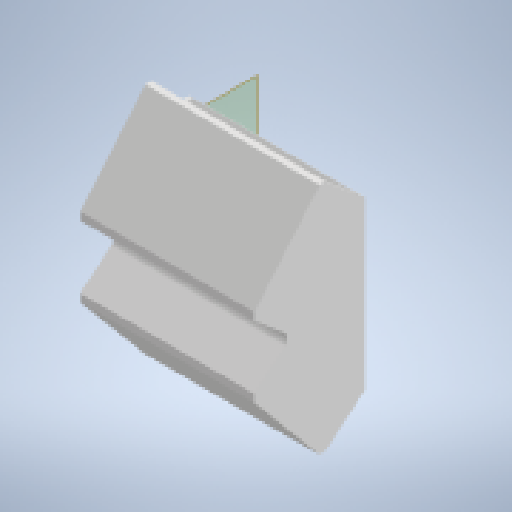
# Autodesk Inventor part: BatterMountv1
Saved by Autodesk Inventor 2023 (Build 270158030, 158C)
## iProperties
Created: 2024-03-25
Part Number: BatterMountv1
Material: Generic
Document SubType Name: Modeling
Designer: lvrectanus0
Density: 1 g/cm^3
Appearance: Default
Author: lvrectanus0
Autodesk Inventor part; units mm, degrees
ref_plane "YZ Plane" through (0, 0, 0) normal (1, 0, 0) x (0, 1, 0)
ref_plane "XZ Plane" through (0, 0, 0) normal (0, 1, 0) x (-1, 0, 0)
ref_plane "XY Plane" through (0, 0, 0) normal (0, 0, 1) x (1, 0, 0)
ref_plane "Work Plane1" through (-37.1475, -26.67, 0) normal (-1, 0, 0) x (0, 0, 1)
sketch "Sketch1" plane through (-37.1475, -26.67, 0) normal (-1, 0, 0) x (0, 0, 1)
  line L0 (-8, 23.8125) -> (-8, 9.525) projected
  line L1 (-8, 9.525) -> (-20.7, 9.525) projected
  ellipse E0 centre (-20.7, 16.6688) end of major axis (-20.7, 23.8125) minor radius 2.54 (-20.7, 23.8125) -> (-20.7, 9.525) ccw projected
  line L2 (-20.7, 23.8125) -> (-8, 23.8125) projected
  ellipse E1 centre (-20.7, 45.2438) end of major axis (-20.7, 50.8) minor radius 2.54 (-20.7, 50.8) -> (-20.7, 39.6875) ccw projected
  line L3 (-20.7, 50.8) -> (-8, 50.8) projected
  line L4 (-8, 50.8) -> (-8, 39.6875) projected
  line L5 (-8, 39.6875) -> (-20.7, 39.6875) projected
  line L6 (0, 53.34) -> (0, 0) projected
  line L7 (0, 53.34) -> (-27.05, 53.34) projected
  line L8 (-27.05, 0) -> (-27.05, 53.34) projected
  line L9 (0, 0) -> (-27.05, 0) projected
  line L10 (0, 0) -> (0, -8.89)
  line L11 (0, -8.89) -> (17.0253, -23.176)
  line L12 (17.0253, -23.176) -> (19.5653, -23.176)
  line L13 (19.5653, -23.176) -> (47.3209, 9.9018)
  line L14 (19.5653, -23.176) -> (62.7453, -23.176) construction
  line L15 (47.3209, 9.9018) -> (47.3209, 12.4418)
  line L16 (47.3209, 12.4418) -> (30.2956, 26.7278) construction
  line L17 (0, -8.89) -> (29.8869, 26.7278) construction
  line L18 (0, -8.89) -> (46.4957, -8.89) construction
  line L19 (30.2956, 26.7278) -> (29.8869, 26.7278) construction
  line L20 (0, 26.67) -> (56.4036, 26.67) construction
  line L21 (47.3209, 12.4418) -> (47.3209, 26.67)
  line L22 (0, 0) -> (0, 26.67)
  line L23 (0, 53.34) -> (0, 62.23)
  line L24 (0, 62.23) -> (17.0253, 76.516)
  line L25 (17.0253, 76.516) -> (19.5653, 76.516)
  line L26 (19.5653, 76.516) -> (47.3209, 43.4382)
  line L27 (19.5653, 76.516) -> (62.7453, 76.516) construction
  line L28 (47.3209, 43.4382) -> (47.3209, 40.8982)
  line L29 (47.3209, 40.8982) -> (30.2956, 26.6122) construction
  line L30 (0, 62.23) -> (29.8869, 26.6122) construction
  line L31 (0, 62.23) -> (46.4957, 62.23) construction
  line L32 (30.2956, 26.6122) -> (29.8869, 26.6122) construction
  line L33 (47.3209, 40.8982) -> (47.3209, 26.67)
  line L34 (0, 53.34) -> (0, 26.67)
  dimension "d0" = 8.89
  dimension "d1" = 22.225
  dimension "d2" = 130
  dimension "d3" = 2.54
  dimension "d4" = 43.18
  dimension "d5" = 50
  dimension "d6" = 2.54
  dimension "d7" = 140
  dimension "d9" = 130
  dimension "d10" = 50
  constraints: 50 end point, 9 symmetric about line, 5 horizontal, 3 equal length, 3 vertical, 2 perpendicular, 1 horizontal alignment, 1 point on line, 2 other
  measures "d0" distance of L6.end L10.end
  measures "d1" distance of L10.end L11.end
  measures "d2" angle of L11 L10
  measures "d3" distance of L11.end L12.end
  measures "d4" distance of L12.end L13.end
  measures "d5" angle of L14 L13
  measures "d6" distance of L13.end L15.end
  measures "d7" angle of L15 L13
  measures "d9" angle of L16 L15
  measures "d10" angle of L18 L17
ref_plane "Work Plane2" through (37.1475, -26.67, -27.05) normal (1, 0, 0) x (0, 1, 0)
extrude "Extrusion1" add sketch "Sketch1" against normal up to surface (74.295 mm away) contours L23 L24 L25 L26 L28 L33 L21 L15 L13 L12 L11 L10 L6
sketch "Sketch2" plane through (-37.1475, -49.846, 17.0253) normal (0, -0.7660444, -0.6427876) x (1, 0, 0)
  line L0 (74.295, -22.225) -> (74.295, 0) projected
  line L1 (0, 0) -> (74.295, 0) projected
  line L2 (0, -22.225) -> (0, 0) projected
  line L3 (0, -22.225) -> (74.295, -22.225) projected
  line L4 (72.7075, -20.6375) -> (72.7075, -1.5875)
  line L5 (72.7075, -1.5875) -> (1.5875, -1.5875)
  line L6 (1.5875, -1.5875) -> (1.5875, -20.6375)
  line L7 (1.5875, -20.6375) -> (72.7075, -20.6375)
  point P0 (37.1475, -45.0825)
  dimension "d13" = 19.05
  constraints: 8 end point, 3 other
  measures "d13" distance between parallel lines of L5 L7
sketch "Sketch3" plane through (-37.1475, 35.56, 0) normal (0, 0.7660444, -0.6427876) x (1, 0, 0)
  line L0 (74.295, -22.225) -> (74.295, 0) projected
  line L1 (0, 0) -> (74.295, 0) projected
  line L2 (0, -22.225) -> (0, 0) projected
  line L3 (0, -22.225) -> (74.295, -22.225) projected
  line L4 (72.7075, -1.5875) -> (72.7075, -20.6375)
  line L5 (72.7075, -20.6375) -> (1.5875, -20.6375)
  line L6 (1.5875, -20.6375) -> (1.5875, -1.5875)
  line L7 (1.5875, -1.5875) -> (72.7075, -1.5875)
  point P0 (37.1475, 22.8575)
  dimension "d14" = 19.05
  constraints: 8 end point, 3 other
  measures "d14" distance between parallel lines of L5 L7
extrude "Extrusion2" cut sketch "Sketch2" against normal blind 44.45 contours L7 L6 L5 L4
extrude "Extrusion3" cut sketch "Sketch3" against normal blind 44.45 contours L4 L5 L6 L7
sketch "Sketch4" plane through (-37.1475, -26.67, 0) normal (-1, 0, 0) x (0, 0, 1)
  line L0 (19.5653, -23.176) -> (47.3209, 9.9018) projected
  line L1 (47.3209, 43.4382) -> (19.5653, 76.516) projected
  line L2 (19.5653, -23.176) -> (47.3209, 9.9018) projected
  line L3 (47.3209, 43.4382) -> (19.5653, 76.516) projected
  line L4 (0, -8.89) -> (17.0253, -23.176) projected
  line L5 (17.0253, -23.176) -> (19.5653, -23.176) projected
  line L6 (19.5653, -23.176) -> (47.3209, 9.9018) projected
  line L7 (47.3209, 9.9018) -> (47.3209, 43.4382) projected
  line L8 (47.3209, 43.4382) -> (19.5653, 76.516) projected
  line L9 (19.5653, 76.516) -> (17.0253, 76.516) projected
  line L10 (17.0253, 76.516) -> (0, 62.23) projected
  line L11 (0, 62.23) -> (0, -8.89) projected
  line L12 (1.2161, -9.9104) -> (15.8092, -22.1555) projected
  line L13 (1.2161, -9.9104) -> (29.788, 24.1403) projected
  line L14 (29.788, 24.1403) -> (44.3812, 11.8951) projected
  line L15 (15.8092, -22.1555) -> (44.3812, 11.8951) projected
  line L16 (15.8092, 75.4955) -> (1.2161, 63.2504) projected
  line L17 (15.8092, 75.4955) -> (44.3812, 41.4449) projected
  line L18 (44.3812, 41.4449) -> (29.788, 29.1997) projected
  line L19 (1.2161, 63.2504) -> (29.788, 29.1997) projected
  line L20 (47.3209, 9.9018) -> (27.3374, 26.67)
  line L21 (27.3374, 26.67) -> (47.3209, 43.4382)
  line L22 (47.3209, 13.2176) -> (31.2889, 26.67)
  line L23 (31.2889, 26.67) -> (47.3209, 40.1224)
  line L24 (47.3209, 9.9018) -> (47.3209, 43.4382) projected
  line L25 (47.3209, 9.9018) -> (47.3209, 43.4382)
  point P0 (0, 26.67)
  point P1 (47.3209, 26.67)
  point P2 (47.3209, 26.67)
  point P3 (47.3209, 13.2176)
  dimension "d20" = 2.54
  constraints: 10 end point, 2 horizontal alignment, 2 midpoint, 2 point on line, 1 collinear, 1 parallel, 1 other
  measures "d20" distance between parallel lines of L20 L22
extrude "Extrusion4" cut sketch "Sketch4" against normal through all contours L22 L23 L7
fillet "Fillet1" radius 3.175 1 edges at (0, 0, 31.2889)
sketch "Sketch5" plane through (-37.1475, -35.56, 0) normal (0, 0, -1) x (-1, 0, 0)
  line L0 (-68.8975, 30.575) -> (-72.7075, 30.575) projected
  arc A0 (-68.8975, 22.765) -> (-68.8975, 30.575) centre (-68.8975, 26.67) ccw projected
  line L1 (-72.7075, 22.765) -> (-68.8975, 22.765) projected
  line L2 (-72.7075, 22.765) -> (-72.7075, 8.89) projected
  arc A1 (-72.7075, 8.89) -> (-71.4375, 7.62) centre (-71.4375, 8.89) ccw projected
  line L3 (-71.4375, 7.62) -> (-22.0025, 7.62) projected
  line L4 (-22.0025, 11.43) -> (-22.0025, 7.62) projected
  arc A2 (-14.1925, 11.43) -> (-22.0025, 11.43) centre (-18.0975, 11.43) ccw projected
  line L5 (-14.1925, 7.62) -> (-14.1925, 11.43) projected
  line L6 (-14.1925, 7.62) -> (-2.8575, 7.62) projected
  arc A3 (-2.8575, 7.62) -> (-1.5875, 8.89) centre (-2.8575, 8.89) ccw projected
  line L7 (-1.5875, 8.89) -> (-1.5875, 62.23) projected
  arc A4 (-1.5875, 62.23) -> (-2.8575, 63.5) centre (-2.8575, 62.23) ccw projected
  line L8 (-2.8575, 63.5) -> (-12.9225, 63.5) projected
  line L9 (-12.9225, 59.69) -> (-12.9225, 63.5) projected
  arc A5 (-20.7325, 59.69) -> (-12.9225, 59.69) centre (-16.8275, 59.69) ccw projected
  line L10 (-20.7325, 63.5) -> (-20.7325, 59.69) projected
  line L11 (-20.7325, 63.5) -> (-71.4375, 63.5) projected
  arc A6 (-71.4375, 63.5) -> (-72.7075, 62.23) centre (-71.4375, 62.23) ccw projected
  line L12 (-72.7075, 62.23) -> (-72.7075, 58.515) projected
  line L13 (-68.8975, 58.515) -> (-72.7075, 58.515) projected
  arc A7 (-68.8975, 50.705) -> (-68.8975, 58.515) centre (-68.8975, 54.61) ccw projected
  line L14 (-72.7075, 50.705) -> (-68.8975, 50.705) projected
  line L15 (-72.7075, 50.705) -> (-72.7075, 30.575) projected
  circle A8 centre (-18.0975, 11.43) radius 2 projected
  circle A9 centre (-68.8975, 26.67) radius 2 projected
  circle A10 centre (-68.8975, 54.61) radius 2 projected
  circle A11 centre (-16.8275, 59.69) radius 2 projected
  point P0 (-37.1475, 35.56)
extrude "Extrusion5" cut sketch "Sketch5" against normal blind 5.8 contours A8 | A9 | A10 | A11
sketch "Sketch6" plane through (-37.1475, -26.67, 0) normal (-1, 0, 0) x (0, 0, 1)
  line L0 (15.8092, -22.1555) -> (1.2161, -9.9104) projected
  line L1 (1.2161, -9.9104) -> (29.788, 24.1403) projected
  arc A0 (15.8092, -22.1555) -> (1.2161, -9.9104) centre (3.1131, -22.468) ccw
  line L2 (1.2161, 63.2504) -> (29.788, 29.1997) projected
  line L3 (15.8092, 75.4955) -> (44.3812, 41.4449) projected
  arc A1 (1.2161, 63.2504) -> (15.8092, 75.4955) centre (3.1131, 75.808) ccw
  line L4 (15.8092, 75.4955) -> (1.2161, 63.2504) projected
  point P0 (0, 26.67)
  dimension "d26" = 12.7
  dimension "d27" = 12.7
  constraints: 4 point on circle, 2 centre point
  measures "d26" radius of A0
  measures "d27" radius of A1
extrude "Extrusion6" cut sketch "Sketch6" against normal up to surface (1.5875 mm away)
sketch "Sketch7" plane through (-37.1475, -26.67, 0) normal (-1, 0, 0) x (0, 0, 1)
  arc A0 (1.2161, 63.2504) -> (15.8092, 75.4955) centre (3.1131, 75.808) ccw projected
  line L0 (1.2161, 63.2504) -> (0, 62.23) projected
  line L1 (0, 62.23) -> (0, -8.89) projected
  line L2 (0, -8.89) -> (1.2161, -9.9104) projected
  arc A1 (15.8092, -22.1555) -> (1.2161, -9.9104) centre (3.1131, -22.468) ccw projected
  line L3 (15.8092, -22.1555) -> (17.0253, -23.176) projected
  line L4 (17.0253, -23.176) -> (19.5653, -23.176) projected
  line L5 (19.5653, -23.176) -> (47.3209, 9.9018) projected
  line L6 (47.3209, 9.9018) -> (47.3209, 13.2176) projected
  line L7 (47.3209, 13.2176) -> (34.1875, 24.2378) projected
  arc A2 (34.1875, 29.1022) -> (34.1875, 24.2378) centre (36.2284, 26.67) ccw projected
  line L8 (34.1875, 29.1022) -> (47.3209, 40.1224) projected
  line L9 (47.3209, 40.1224) -> (47.3209, 43.4382) projected
  line L10 (47.3209, 43.4382) -> (19.5653, 76.516) projected
  line L11 (19.5653, 76.516) -> (17.0253, 76.516) projected
  line L12 (17.0253, 76.516) -> (15.8092, 75.4955) projected
  line L13 (0.3078, 54.17) -> (0.3078, -0.83) projected
  line L14 (6.35, -0.83) -> (0.3078, -0.83) projected
  line L15 (6.35, 54.17) -> (6.35, -0.83) projected
  line L16 (0.3078, 54.17) -> (6.35, 54.17) projected
  line L17 (17.0253, 76.516) -> (0, 62.23) projected
  line L18 (0, 62.23) -> (6.35, 62.23)
  line L19 (6.35, 62.23) -> (6.35, 55.88)
  line L20 (6.35, 55.88) -> (0, 55.88)
  line L21 (0, 55.88) -> (0, 62.23)
  line L22 (47.3209, 43.4382) -> (19.5653, 76.516) projected
  line L23 (24.4634, 70.6787) -> (19.599, 66.597)
  line L24 (19.599, 66.597) -> (23.6807, 61.7326)
  line L25 (23.6807, 61.7326) -> (28.5451, 65.8143)
  line L26 (24.4634, 70.6787) -> (28.5451, 65.8143)
  line L27 (42.4229, 49.2754) -> (37.5585, 45.1937)
  line L28 (37.5585, 45.1937) -> (33.4768, 50.0581)
  line L29 (33.4768, 50.0581) -> (38.3412, 54.1398)
  line L30 (42.4229, 49.2754) -> (38.3412, 54.1398)
  line L31 (36.2284, 26.67) -> (0, 26.67) construction
  arc A3 (15.8092, -22.1555) -> (1.2161, -9.9104) centre (3.1131, -22.468) ccw
  line L32 (1.2161, -9.9104) -> (0, -8.89)
  line L33 (47.3209, 9.9018) -> (19.5653, -23.176)
  line L34 (19.5653, -23.176) -> (17.0253, -23.176)
  line L35 (17.0253, -23.176) -> (15.8092, -22.1555)
  line L36 (0.3078, -0.83) -> (6.35, -0.83)
  line L37 (17.0253, -23.176) -> (0, -8.89)
  line L38 (0, -8.89) -> (6.35, -8.89)
  line L39 (6.35, -8.89) -> (6.35, -2.54)
  line L40 (6.35, -2.54) -> (0, -2.54)
  line L41 (0, -2.54) -> (0, -8.89)
  line L42 (47.3209, 9.9018) -> (19.5653, -23.176)
  line L43 (24.4634, -17.3387) -> (19.599, -13.257)
  line L44 (19.599, -13.257) -> (23.6807, -8.3926)
  line L45 (23.6807, -8.3926) -> (28.5451, -12.4743)
  line L46 (24.4634, -17.3387) -> (28.5451, -12.4743)
  line L47 (42.4229, 4.0646) -> (37.5585, 8.1463)
  line L48 (37.5585, 8.1463) -> (33.4768, 3.2819)
  line L49 (33.4768, 3.2819) -> (38.3412, -0.7998)
  line L50 (42.4229, 4.0646) -> (38.3412, -0.7998)
  circle A4 centre (3.3289, 13.97) radius 2 projected
  circle A5 centre (3.3289, 39.37) radius 2 projected
  point P0 (0, 55.88)
  point P1 (24.4634, -17.3387)
  point P2 (0, -2.54)
  dimension "d30" = 6.35
  dimension "d31" = 6.35
  dimension "d34" = 6.35
  dimension "d35" = 7.62
  dimension "d36" = 6.35
  dimension "d37" = 6.35
  dimension "d38" = 7.62
  constraints: 64 end point, 12 symmetric about line, 8 point on line, 7 perpendicular, 5 parallel, 2 horizontal, 2 point on circle, 1 centre point, 1 collinear, 1 other
  measures "d30" distance of L19.end L20.end
  measures "d31" distance of L18.end L19.end
  measures "d34" distance of L23.start L23.end
  measures "d35" distance of L10.end L23.start
  measures "d36" distance of L23.end L24.end
  measures "d37" distance of L27.end L28.end
  measures "d38" distance of L27.start L9.end
extrude "Extrusion7" add sketch "Sketch7" along normal blind 6.35 contours L18 L19 L20 L1 | L40 L39 L38 L1 | L10 L25 L24 L23 | L10 L27 L28 L29 | L43 L44 L45 L5 | L49 L48 L47 L5
chamfer "Chamfer1" distance 6.35 angle 45 13 edges at (-37.1475, 20.5646, 39.9907) (-37.1475, 37.1035, 26.1129) (-37.1475, -25.4289, 35.909) (-37.1475, -41.9678, 22.0312) (-37.1475, -37.4948, 21.6398) (-37.1475, -20.9559, 35.5176) (-37.1475, -20.5646, 39.9907) (-37.1475, 20.9559, 35.5176) (-37.1475, 25.4289, 35.909) (-37.1475, 41.9678, 22.0312) (-37.1475, 37.4948, 21.6398) (-37.1475, 32.385, 6.35) (-37.1475, -32.385, 6.35)
sketch "Sketch8" plane through (-43.4975, -26.67, 0) normal (-1, 0, 0) x (0, 0, 1)
  line L0 (6.35, -2.54) -> (0, -2.54) construction
  line L1 (0, -2.54) -> (0, -8.89) construction
  line L2 (0, -8.89) -> (6.35, -8.89) construction
  line L3 (6.35, -8.89) -> (6.35, -2.54) construction
  line L4 (19.599, -13.257) -> (24.4634, -17.3387) construction
  line L5 (24.4634, -17.3387) -> (28.5451, -12.4743) construction
  line L6 (28.5451, -12.4743) -> (23.6807, -8.3926) construction
  line L7 (23.6807, -8.3926) -> (19.599, -13.257) construction
  line L8 (33.4768, 3.2819) -> (38.3412, -0.7998) construction
  line L9 (38.3412, -0.7998) -> (42.4229, 4.0646) construction
  line L10 (42.4229, 4.0646) -> (37.5585, 8.1463) construction
  line L11 (37.5585, 8.1463) -> (33.4768, 3.2819) construction
  line L12 (37.5585, 45.1937) -> (42.4229, 49.2754) construction
  line L13 (42.4229, 49.2754) -> (38.3412, 54.1398) construction
  line L14 (38.3412, 54.1398) -> (33.4768, 50.0581) construction
  line L15 (33.4768, 50.0581) -> (37.5585, 45.1937) construction
  line L16 (23.6807, 61.7326) -> (28.5451, 65.8143) construction
  line L17 (28.5451, 65.8143) -> (24.4634, 70.6787) construction
  line L18 (24.4634, 70.6787) -> (19.599, 66.597) construction
  line L19 (19.599, 66.597) -> (23.6807, 61.7326) construction
  line L20 (6.35, 62.23) -> (0, 62.23) construction
  line L21 (0, 62.23) -> (0, 55.88) construction
  line L22 (0, 55.88) -> (6.35, 55.88) construction
  line L23 (6.35, 55.88) -> (6.35, 62.23) construction
  line L24 (0, -2.54) -> (0, -8.89) construction
  line L25 (6.35, -2.54) -> (0, -2.54) construction
  line L26 (0, -8.89) -> (6.35, -2.54) construction
  line L27 (0, -8.89) -> (6.35, -8.89) construction
  line L28 (6.35, -2.54) -> (6.35, -8.89) construction
  line L29 (6.35, -8.89) -> (0, -2.54) construction
  line L30 (23.6807, -8.3926) -> (19.599, -13.257) construction
  line L31 (28.5451, -12.4743) -> (19.599, -13.257) construction
  line L32 (24.4634, -17.3387) -> (28.5451, -12.4743) construction
  line L33 (19.599, -13.257) -> (24.4634, -17.3387) construction
  line L34 (24.4634, -17.3387) -> (23.6807, -8.3926) construction
  line L35 (33.4768, 3.2819) -> (42.4229, 4.0646) construction
  line L36 (24.5307, 2.4992) -> (33.4768, 3.2819) construction
  line L37 (37.5585, 8.1463) -> (36.7758, 17.0924) construction
  line L38 (37.5585, 8.1463) -> (38.3412, -0.7998) construction
  line L39 (33.4768, 50.0581) -> (37.5585, 45.1937) construction
  line L40 (42.4229, 49.2754) -> (38.3412, 54.1398) construction
  line L41 (37.5585, 45.1937) -> (38.3412, 54.1398) construction
  line L42 (38.3412, 54.1398) -> (42.4229, 49.2754) construction
  line L43 (42.4229, 49.2754) -> (33.4768, 50.0581) construction
  line L44 (23.6807, 61.7326) -> (28.5451, 65.8143) construction
  line L45 (23.6807, 61.7326) -> (24.4634, 70.6787) construction
  line L46 (19.599, 66.597) -> (12.4699, 67.2207) construction
  line L47 (19.599, 66.597) -> (28.5451, 65.8143) construction
  line L48 (6.35, 62.23) -> (0, 62.23) construction
  line L49 (12.7, 55.88) -> (0, 55.88) construction
  line L50 (6.35, 62.23) -> (0, 55.88) construction
  line L51 (0, 55.88) -> (6.35, 55.88) construction
  line L52 (0, 62.23) -> (6.35, 55.88) construction
  line L53 (6.35, 55.88) -> (6.35, 62.23) construction
  point P0 (0, 26.67)
  point P1 (3.175, -5.715)
  point P2 (24.072, -12.8657)
  point P3 (37.9498, 3.6732)
  point P4 (37.9498, 49.6668)
  point P5 (24.072, 66.2057)
  point P6 (3.175, 59.055)
  constraints: 32 end point, 6 midpoint, 6 perpendicular, 5 collinear, 1 point on line
hole "Hole1" at (-43.4975, -32.385, 3.175) at (-43.4975, -39.5357, 24.072) at (-43.4975, -22.9968, 37.9498) at (-43.4975, 22.9968, 37.9498) at (-43.4975, 39.5357, 24.072) at (-43.4975, 32.385, 3.175) direction (1, 0, 0) diameter 4 depth 5.8
sketch "Sketch9" plane through (37.1475, -35.56, 0) normal (1, 0, 0) x (0, 0, -1)
  line L0 (-23.6807, 70.6226) -> (-28.5451, 74.7043) projected
  line L1 (-28.5451, 74.7043) -> (-24.4634, 79.5687) projected
  line L2 (-24.4634, 79.5687) -> (-19.599, 75.487) projected
  line L3 (-19.599, 75.487) -> (-23.6807, 70.6226) projected
  line L4 (-6.35, 71.12) -> (0, 71.12) projected
  line L5 (0, 71.12) -> (0, 64.77) projected
  line L6 (0, 64.77) -> (-6.35, 64.77) projected
  line L7 (-6.35, 64.77) -> (-6.35, 71.12) projected
  line L8 (-37.5585, 54.0837) -> (-42.4229, 58.1654) projected
  line L9 (-42.4229, 58.1654) -> (-38.3412, 63.0298) projected
  line L10 (-38.3412, 63.0298) -> (-33.4768, 58.9481) projected
  line L11 (-33.4768, 58.9481) -> (-37.5585, 54.0837) projected
  line L12 (-19.599, -4.367) -> (-24.4634, -8.4487) projected
  line L13 (-24.4634, -8.4487) -> (-28.5451, -3.5843) projected
  line L14 (-28.5451, -3.5843) -> (-23.6807, 0.4974) projected
  line L15 (-23.6807, 0.4974) -> (-19.599, -4.367) projected
  line L16 (-6.35, 6.35) -> (0, 6.35) projected
  line L17 (0, 6.35) -> (0, 0) projected
  line L18 (0, 0) -> (-6.35, 0) projected
  line L19 (-6.35, 0) -> (-6.35, 6.35) projected
  line L20 (-33.4768, 12.1719) -> (-38.3412, 8.0902) projected
  line L21 (-38.3412, 8.0902) -> (-42.4229, 12.9546) projected
  line L22 (-42.4229, 12.9546) -> (-37.5585, 17.0363) projected
  line L23 (-37.5585, 17.0363) -> (-33.4768, 12.1719) projected
  circle A0 centre (-3.175, 67.945) radius 2 projected
  circle A1 centre (-24.072, 75.0957) radius 2 projected
  circle A2 centre (-37.9498, 58.5568) radius 2 projected
  circle A3 centre (-37.9498, 12.5632) radius 2 projected
  circle A4 centre (-24.072, -3.9757) radius 2 projected
  circle A5 centre (-3.175, 3.175) radius 2 projected
  point P0 (0, 35.56)
extrude "Extrusion8" add sketch "Sketch9" along normal blind 6.35
chamfer "Chamfer2" distance 6.35 angle 45 14 edges at (37.1475, 41.9678, 22.0312) (37.1475, 37.4948, 21.6398) (37.1475, 32.385, 6.35) (37.1475, 37.1035, 26.1129) (37.1475, 20.5646, 39.9907) (37.1475, -20.5646, 39.9907) (37.1475, -37.1035, 26.1129) (37.1475, -32.385, 6.35) (37.1475, -25.4289, 35.909) (37.1475, -41.9678, 22.0312) (37.1475, 20.9559, 35.5176) (37.1475, 25.4289, 35.909) (37.1475, -37.4948, 21.6398) (37.1475, -20.9559, 35.5176)
sketch "Sketch10" plane through (-37.1475, -26.67, 0) normal (-1, 0, 0) x (0, 0, 1)
  circle A0 centre (3.3289, 13.97) radius 2 projected
  circle A1 centre (25.788, 26.67) radius 2 projected
  circle A2 centre (3.3289, 39.37) radius 2 projected
  point P0 (0, 26.67)
hole "Hole2" at (-37.1475, -12.7, 3.3289) at (-37.1475, 0, 25.788) at (-37.1475, 12.7, 3.3289) direction (1, 0, 0) diameter 4 depth 5.8
sketch "Sketch11" plane through (37.1475, 0, 36.2284) normal (1, 0, 0) x (0, 0, -1)
  circle A0 centre (32.8995, 12.7) radius 2 projected
  circle A1 centre (32.8995, 12.7) radius 2 projected
  circle A2 centre (32.8995, -12.7) radius 2 projected
  circle A3 centre (32.8995, -12.7) radius 2 projected
  circle A4 centre (10.4404, 0) radius 2 projected
  circle A5 centre (10.4404, 0) radius 2 projected
  point P0 (36.2284, 0)
hole "Hole3" at (37.1475, 12.7, 3.3289) at (37.1475, -12.7, 3.3289) at (37.1475, 0, 25.788) direction (-1, 0, 0) diameter 4 depth 5.8
body "Solid1"
